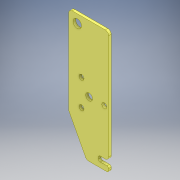
# Autodesk Inventor part: bras_amortisseur
Saved by Autodesk Inventor 2017 (Build 210142000, 142)
## iProperties
Created: 2017-04-12
Part Number: bras_amortisseur
Material: Generic
Document SubType Name: Modeling
Designer: franc
Density: 1 g/cm^3
Appearance: Default
Author: franc
Autodesk Inventor part; units mm, degrees
ref_plane "YZ Plane" through (0, 0, 0) normal (1, 0, 0) x (0, 1, 0)
ref_plane "XZ Plane" through (0, 0, 0) normal (0, 1, 0) x (-1, 0, 0)
ref_plane "XY Plane" through (0, 0, 0) normal (0, 0, 1) x (1, 0, 0)
sketch "Sketch1" plane through (0, 0, 0) normal (0, 1, 0) x (-1, 0, 0)
  line L0 (4.5998, 20.0337) -> (-14.9002, 20.0337)
  line L1 (6.3706, -32.4029) -> (-3.3383, -50.8959)
  line L2 (6.5998, -31.4732) -> (6.5998, 18.0337)
  line L3 (-5.1091, -51.9663) -> (-14.9002, -51.9663)
  circle A0 centre (1.5998, 15.0337) radius 2.5
  circle A1 centre (-5.4002, -18.9663) radius 2
  line L4 (-14.9002, -45.9663) -> (-12.597, -45.9663)
  line L5 (-12.0688, -48.9663) -> (-14.0688, -48.9663)
  line L6 (-16.9002, 18.0337) -> (-16.9002, -43.9663)
  arc A2 (-16.9002, -43.9663) -> (-14.9002, -45.9663) centre (-14.9002, -43.9663) ccw
  arc A3 (-5.1091, -51.9663) -> (-3.3383, -50.8959) centre (-5.1091, -49.9663) ccw
  arc A4 (6.3706, -32.4029) -> (6.5998, -31.4732) centre (4.5998, -31.4732) ccw
  arc A5 (6.5998, 18.0337) -> (4.5998, 20.0337) centre (4.5998, 18.0337) ccw
  arc A6 (-14.9002, 20.0337) -> (-16.9002, 18.0337) centre (-14.9002, 18.0337) ccw
  circle A7 centre (-14.4002, -18.9663) radius 1.5
  circle A8 centre (-0.9002, -11.172) radius 1.5
  circle A9 centre (-0.9002, -26.7605) radius 1.5
  line L7 (-12.597, -45.9663) -> (-11.9002, -45.9663)
  line L8 (-10.9002, -46.9663) -> (-10.9002, -47.9663)
  line L9 (-12.3368, -48.9663) -> (-11.9002, -48.9663)
  line L10 (-14.9002, -51.9663) -> (-15.9002, -51.9663)
  line L11 (-16.9002, -50.9663) -> (-16.9002, -49.9663)
  line L12 (-15.9002, -48.9663) -> (-14.0688, -48.9663)
  arc A10 (-10.9002, -46.9663) -> (-11.9002, -45.9663) centre (-11.9002, -46.9663) ccw
  arc A11 (-11.9002, -48.9663) -> (-10.9002, -47.9663) centre (-11.9002, -47.9663) ccw
  arc A12 (-15.9002, -48.9663) -> (-16.9002, -49.9663) centre (-15.9002, -49.9663) ccw
  arc A13 (-16.9002, -50.9663) -> (-15.9002, -51.9663) centre (-15.9002, -50.9663) ccw
  point P0 (0, 0)
  point P1 (6.5998, 20.0337)
  point P2 (-16.9002, 20.0337)
  point P3 (6.5998, -31.9663)
  point P4 (-3.9002, -51.9663)
  point P5 (-16.9002, -45.9663)
  point P6 (-10.9002, -45.9663)
  point P7 (-10.9002, -48.9663)
  point P8 (-16.9002, -51.9663)
  point P9 (-16.9002, -48.9663)
  dimension "d1" = 23.5
  dimension "d3" = 52
  dimension "d5" = 5
  dimension "d6" = 5
  dimension "d7" = 5
  dimension "d8" = 4
  dimension "d9" = 12
  dimension "d10" = 39
  dimension "d28" = 3
  dimension "d29" = 9
  dimension "d30" = 2.5
  dimension "d31" = 3
  dimension "d32" = 3
  dimension "d33" = 120
  dimension "d34" = 120
  dimension "d35" = 9
  dimension "d36" = 9
  dimension "d37" = 3
  dimension "d38" = 6
  dimension "d39" = 3
  dimension "d40" = 6
  dimension "d41" = 1
  constraints: 26 end point, 19 point on line, 18 point on circle, 18 tangent, 14 centre point, 5 equal radius, 5 horizontal, 4 perpendicular, 2 vertical, 1 parallel
  measures "d1" distance of point (6.6, 20.034) point (-16.9, 20.034)
  measures "d3" distance of point (6.6, -31.966) point (6.6, 20.034)
  measures "d5" distance from line of A0.centre L2
  measures "d6" distance from line of L0 A0.centre
  measures "d7" diameter of A0
  measures "d8" diameter of A1
  measures "d9" distance from line of L2 A1.centre
  measures "d10" distance from line of L0 A1.centre
  measures "d28" diameter of A7
  measures "d29" distance of A7.centre A1.centre
  measures "d30" distance from line of L6 A7.centre
  measures "d31" diameter of A8
  measures "d32" diameter of A9
  measures "d35" distance of A8.centre A1.centre
  measures "d36" distance of A9.centre A1.centre
  measures "d37" distance of point (-10.9, -45.966) point (-10.9, -48.966)
  measures "d38" distance between parallel lines of L6 L8
  measures "d39" distance of point (-16.9, -51.966) point (-16.9, -48.966)
  measures "d40" distance between parallel lines of L11 L8
  measures "d41" radius of A10
extrude "Extrusion1" add sketch "Sketch1" along normal blind 1.5
body "Solid1"
